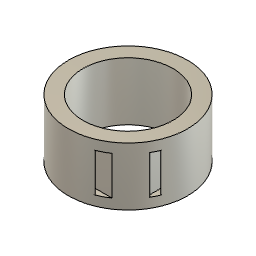
Encoder_Ring (Autodesk Fusion 360 design; units mm, degrees)
Autodesk Fusion 360 part; units mm, degrees
sketch "Sketch1" plane through (0, 0, 0) normal (0, 1, 0) x (1, 0, 0)
  circle A0 centre (0, 0) radius 12.3
  circle A1 centre (0, 0) radius 9.3
  dimension "d1" = 24.6
  dimension "d2" = 3
  constraint coincident A0.centre A1.centre
  measures "d1" diameter of A0
  measures "d2" distance of A0 A1
extrude "Extrude1" add sketch "Sketch1" along normal blind 12
sketch "Sketch2" plane through (0, 0, 0) normal (0, 0, 1) x (1, 0, 0)
  line L0 (10.2, 10) -> (11.4, 10)
  line L1 (11.4, 10) -> (11.4, 2)
  line L2 (11.4, 2) -> (10.2, 2)
  line L3 (10.2, 2) -> (10.2, 10)
  line L4 (10.2, 2) -> (11.4, 10) construction
  line L5 (12.3, 12) -> (-12.3, 12) construction
  line L6 (-9.3, 0) -> (9.3, 0) construction
  line L7 (9.3, 0) -> (12.3, 12) construction
  point P0 (10.8, 6)
  dimension "d5" = 1.2
  dimension "d6" = 8
  constraint horizontal L0
  constraint vertical L1
  constraint horizontal L2
  constraint vertical L3
  constraint midpoint L4 P0
  constraint coincident L6.end L7.start
  constraint coincident L5.start L7.end
  constraint midpoint P0 L7
  measures "d5" distance of L1 L3
  measures "d6" distance of L0.end L1.end
ref_plane "WorkPlane1" through (0, 6, 0) normal (0, 1, 0) x (0, 0, 1)
sketch "Sketch3" plane through (0, 6, 0) normal (0, 1, 0) x (1, 0, 0)
  line L0 (10.8, 0) -> (10.8, -6.15)
  line L1 (0, 0) -> (0, -12.3) construction
  circle A0 centre (0, 0) radius 12.3 construction
  circle A1 centre (0, 0) radius 9.3 construction
  arc A2 (10.8, 0) -> (0, -10.8) centre (0, 0) ccw
  line L2 (0, -10.8) -> (10.8, -10.8)
  point P0 (10.8, 0)
  point P1 (0, -6.15)
  point P2 (0, -10.3)
  constraint vertical L0
  constraint coincident P0 L0.start
  constraint coincident L1.start A0.centre
  constraint vertical L1
  constraint coincident L1.end A0
  constraint midpoint P1 L1
  constraint horizontal L0.end P1
  constraint coincident L1 P2
  constraint concentric A1 A2
  constraint coincident P0 A2
  constraint coincident L1 A2.end
  constraint tangent A2 L2
  constraint coincident L0 L2.end
sweep "Sweep1" cut profiles "Sketch2" path "Sketch3" along L2 A2 L0 section 1
